# Autodesk Inventor part: Welle
Saved by Autodesk Inventor 2016 (Build 200138000, 138)
## iProperties
Created: 2014-12-19
Part Number: Welle
Material: Steel
Document SubType Name: Modeling
Designer: 4ndreas
Density: 7.85 g/cm^3
Appearance: Steel
Mass: 11.1408 g
Surface Area: 10.2953 cm^2
Volume: 1.41921 cm^3
CustomPartVersion: 1
Author: 4ndreas
Autodesk Inventor part; units mm, degrees
ref_plane "Startebene" through (0, 0, 0) normal (1, 0, 0) x (0, 1, 0)
ref_plane "XZ Plane" through (0, 0, 0) normal (0, 1, 0) x (-1, 0, 0)
ref_plane "XY Plane" through (0, 0, 0) normal (0, 0, 1) x (1, 0, 0)
sketch "Hauptskizze" plane through (0, 0, 0) normal (0, 0, 1) x (1, 0, 0)
  line L0 (0, 0) -> (55, 0)
  line L1 (0, 0) -> (0, 3)
  line L2 (40, 3) -> (40, 2.5)
  line L3 (0, 3) -> (40, 3)
  line L4 (55, 2.5) -> (55, 0)
  line L5 (40, 2.5) -> (55, 2.5)
  dimension "d3" = 6
  dimension "d14" = 5
  constraints: 12 end point, 3 horizontal, 3 vertical
  measures "d3" diameter of L3 L0
  measures "d14" diameter of L5 L0
revolve "Umdrehung1" add sketch "Hauptskizze" angle 360 about axis through (0, 0, 0) along (1, 0, 0)
chamfer "Fase4" distance 0.5 angle 45 1 edges at (0, -3, 0) measured on face at (13.3333, 2.9612, -0.4812)
chamfer "Fase5" distance 0.5 angle 45 1 edges at (55, -2.5, 0) measured on face at (45, 2.4919, -0.2012)
chamfer "Fase3" [suppressed]
chamfer "Fase2" distance 0.5 angle 45 1 edges at (40, -3, 0) measured on face at (13.6667, 2.9903, -0.2414)
